Autodesk Inventor part; units mm, degrees
(part 2 of 2)
sketch "Boceto3" plane through (0, 2, 0) normal (0, 1, 0) x (1, 0, 0)
  line L0 (35.7041, 64.3419) -> (35.7041, 63.6919)
  line L1 (35.7042, 59.1622) -> (35.7042, 59.8122)
  line L2 (37.6679, 61.7621) -> (37.6747, 62.4121)
  line L3 (37.6747, 62.4121) -> (38.9746, 62.3985)
  line L4 (37.6679, 61.7621) -> (37.6612, 61.1121)
  line L5 (37.6612, 61.1121) -> (38.961, 61.0986)
  line L6 (41.5539, 61.0919) -> (42.8539, 61.0919) construction
  line L7 (42.8539, 61.0919) -> (42.8539, 58.4716) construction
  spline S0 degree 2 poles (41.5539, 61.0919) (42.8539, 61.0919) (42.8539, 58.4716) knots 1 1 1 2 2 2
  line L8 (41.554, 62.3716) -> (44.1539, 62.3716) construction
  line L9 (44.1539, 62.3716) -> (44.1539, 58.4716) construction
  spline S1 degree 2 poles (41.554, 62.3716) (44.1539, 62.3716) (44.1539, 58.4716) knots 1 1 1 2 2 2
  line L10 (38.954, 61.0919) -> (41.554, 61.0919)
  line L11 (38.9541, 62.3919) -> (41.554, 62.3716)
  line L12 (37.6542, 60.4419) -> (35.7042, 60.4622)
  line L13 (37.6813, 63.0419) -> (35.7041, 63.0419)
  line L14 (37.6813, 63.0419) -> (37.6747, 62.4121)
  line L15 (37.6612, 61.1121) -> (37.6542, 60.4419)
  line L16 (42.8539, 57.8216) -> (44.1539, 57.8216)
  line L17 (44.1539, 57.8216) -> (44.1539, 58.4716)
  line L18 (44.1539, 57.8216) -> (43.8939, 57.8216)
  line L19 (42.8539, 58.4716) -> (42.8539, 57.8216)
  line L20 (58.9613, 57.27) -> (63.5735, 61.1094)
  line L21 (64.2117, 60.8104) -> (64.2117, 53.2631)
  line L22 (58.9754, 56.8292) -> (63.5531, 52.9999)
  arc A0 (63.5531, 52.9999) -> (64.2117, 53.2631) centre (63.7962, 53.3472) ccw
  arc A1 (64.2117, 60.8104) -> (63.5735, 61.1094) centre (63.7975, 60.7568) ccw
  arc A2 (58.9613, 57.27) -> (58.9754, 56.8292) centre (59.2258, 57.0578) ccw
  line L23 (64.4328, 57.3171) -> (69.0449, 61.1564)
  line L24 (69.6831, 60.8575) -> (69.6831, 53.3101)
  line L25 (64.4468, 56.8762) -> (69.0245, 53.0469)
  arc A3 (69.0245, 53.0469) -> (69.6831, 53.3101) centre (69.2676, 53.3943) ccw
  arc A4 (69.6831, 60.8575) -> (69.0449, 61.1564) centre (69.2689, 60.8039) ccw
  arc A5 (64.4328, 57.3171) -> (64.4468, 56.8762) centre (64.6972, 57.1049) ccw
  line L26 (58.9613, 57.27) -> (63.5735, 61.1094)
  line L27 (64.2117, 60.8104) -> (64.2117, 53.2631)
  line L28 (58.9754, 56.8292) -> (63.5531, 52.9999)
  arc A6 (58.9613, 57.27) -> (58.9754, 56.8292) centre (59.2258, 57.0578) ccw
  line L29 (69.6831, 60.8575) -> (69.6831, 53.3101)
  line L30 (64.4328, 57.3171) -> (69.0449, 61.1564)
  line L31 (64.4468, 56.8762) -> (69.0245, 53.0469)
  arc A7 (64.4328, 57.3171) -> (64.4468, 56.8762) centre (64.6972, 57.1049) ccw
  line L32 (128.7561, 56.7254) -> (133.3696, 60.5658)
  line L33 (134.0065, 60.2673) -> (134.0065, 52.7184)
  line L34 (128.7702, 56.2845) -> (133.3479, 52.4552)
  arc A8 (133.3479, 52.4552) -> (134.0065, 52.7184) centre (133.591, 52.8025) ccw
  arc A9 (128.7561, 56.7254) -> (128.7702, 56.2845) centre (129.0205, 56.5132) ccw
  line L35 (139.4779, 60.3128) -> (139.4779, 52.7655)
  arc A10 (138.8193, 52.5023) -> (139.4779, 52.7655) centre (139.0624, 52.8496) ccw
  line L36 (134.2275, 56.7724) -> (138.8397, 60.6118)
  line L37 (134.2416, 56.3316) -> (138.8193, 52.5023)
  arc A11 (134.2275, 56.7724) -> (134.2416, 56.3316) centre (134.4919, 56.5602) ccw
  arc A12 (134.0065, 60.2673) -> (133.3696, 60.5658) centre (133.618, 60.2673) ccw
  arc A13 (139.4779, 60.3128) -> (138.8397, 60.6118) centre (139.0799, 60.294) ccw
  arc A14 (101.959, 62.5573) -> (101.9701, 63.0852) centre (105.955, 62.7371) ccw
  spline S2 degree 3 poles (101.9701, 63.0852) (100.3787, 62.5265) (98.8474, 62.1955) (96.8436, 62.2447) knots 0 0 0 0 1 1 1 1
  circle A15 centre (105.955, 62.7371) radius 1
  arc A16 (108.9509, 62.8921) -> (106.5532, 65.6768) centre (105.955, 62.7371) ccw
  line L38 (109.0736, 62.5385) -> (108.7201, 62.8921)
  line L39 (109.0736, 62.5385) -> (109.4272, 62.8921)
  arc A17 (109.2013, 62.8921) -> (106.5532, 65.9316) centre (105.955, 62.7371) ccw
  line L40 (109.4272, 62.8921) -> (109.2013, 62.8921)
  line L41 (108.9509, 62.8921) -> (108.7201, 62.8921)
  line L42 (102.8865, 63.4069) -> (101.0538, 62.7635) construction
  arc A18 (101.233, 62.841) -> (102.6982, 63.3554) centre (94.7176, 83.7432) ccw construction
  line L43 (96.8436, 62.2447) -> (97.002, 61.7463)
  line L44 (106.5532, 65.9316) -> (106.5532, 65.6768)
  line L45 (35.7041, 64.3419) -> (35.7041, 64.4719)
  line L46 (35.7041, 64.3419) -> (35.7041, 65.6419)
  line L47 (35.7041, 65.6419) -> (33.7541, 65.6419)
  line L48 (33.7541, 65.6419) -> (33.7541, 64.3419)
  line L49 (33.7541, 64.3419) -> (22.7041, 64.3419)
  line L50 (22.7041, 59.1419) -> (22.7041, 64.3419)
  line L51 (33.7541, 59.1419) -> (33.7541, 57.8419)
  line L52 (33.7541, 57.8419) -> (35.704, 57.8419)
  line L53 (35.7042, 57.8419) -> (35.7042, 59.1622)
  line L54 (33.7541, 59.1419) -> (22.7041, 59.1419)
  line L55 (103.5, 23.3722) -> (103.5, 22.8472)
  line L56 (103.5, 19.1886) -> (103.5, 19.7136)
  line L57 (105.0751, 20.2386) -> (103.5, 20.2386)
  line L58 (105.075, 22.3222) -> (103.5, 22.3222)
  line L59 (105.075, 22.3222) -> (105.075, 21.83)
  line L60 (105.0751, 20.78) -> (105.0751, 20.2386)
  line L61 (103.5, 23.3722) -> (103.5, 23.4772)
  line L62 (103.5, 23.3722) -> (103.5, 24.4222)
  line L63 (103.5, 24.4222) -> (101.925, 24.4222)
  line L64 (101.925, 24.4222) -> (101.925, 23.3722)
  line L65 (101.925, 23.3722) -> (93, 23.3722)
  line L66 (93, 19.1722) -> (93, 23.3722)
  line L67 (101.925, 19.1722) -> (101.925, 18.1222)
  line L68 (101.925, 18.1222) -> (103.5, 18.1222)
  line L69 (103.5, 18.1222) -> (103.5, 19.1886)
  line L70 (101.925, 19.1722) -> (93, 19.1722)
  line L71 (103.5, 20.2386) -> (103.5, 19.7136)
  line L72 (103.5, 22.3222) -> (103.5, 22.8472)
  line L73 (35.7042, 60.4622) -> (35.7042, 59.8122)
  line L74 (35.7041, 63.6919) -> (35.7041, 63.0419)
  line L75 (105.075, 21.605) -> (104.7751, 21.605)
  line L76 (104.7751, 21.605) -> (104.7751, 21.005)
  line L77 (104.7751, 21.005) -> (105.0751, 21.005)
  line L78 (105.0751, 21.005) -> (105.0751, 20.78)
  line L79 (105.075, 21.83) -> (105.075, 21.605)
  line L80 (67.3453, 22.5754) -> (66.2953, 22.5754)
  line L81 (66.2953, 22.5754) -> (66.2953, 21.8754)
  line L82 (67.3453, 21.8754) -> (67.3453, 22.5754)
  line L83 (67.3453, 21.8754) -> (67.3453, 21.9454)
  line L84 (67.3453, 21.8754) -> (67.3453, 21.5254)
  line L85 (68.3953, 21.1754) -> (67.3453, 21.1754)
  line L86 (68.3953, 19.7739) -> (67.3453, 19.7754)
  line L87 (67.3453, 19.0754) -> (67.3453, 19.4254)
  line L88 (67.3453, 18.3644) -> (67.3453, 19.0754)
  line L89 (66.2953, 19.074) -> (66.2953, 18.374)
  line L90 (66.2953, 18.374) -> (67.3453, 18.374)
  line L91 (68.3953, 20.1348) -> (68.3953, 19.7739)
  line L92 (67.3453, 19.7754) -> (67.3453, 19.4254)
  line L93 (67.3453, 21.1754) -> (67.3453, 21.5254)
  line L94 (68.3953, 20.2848) -> (68.3953, 20.1348)
  line L95 (68.3953, 21.1754) -> (68.3953, 20.7869)
  line L96 (65.2366, 21.874) -> (65.2366, 19.074)
  line L97 (65.2366, 21.8754) -> (66.2953, 21.8754)
  line L98 (65.2366, 19.074) -> (66.2953, 19.074)
  line L99 (122.2298, 31.1299) -> (122.2298, 16.1299)
  line L100 (122.2298, 16.1299) -> (113.2298, 16.1299)
  line L101 (121.2298, 25.6299) -> (121.2298, 21.6299)
  circle A19 centre (120.4673, 19.4799) radius 0.45
  circle A20 centre (118.8673, 19.4799) radius 0.45
  circle A21 centre (117.2673, 19.4799) radius 0.45
  circle A22 centre (118.8673, 24.2799) radius 0.45
  circle A23 centre (120.4673, 24.2799) radius 0.45
  circle A24 centre (117.2673, 24.2799) radius 0.45
  circle A25 centre (118.8673, 29.0799) radius 0.45
  circle A26 centre (120.4673, 29.0799) radius 0.45
  circle A27 centre (117.2673, 29.0799) radius 0.45
  line L102 (114.9823, 17.6299) -> (117.0198, 17.6299)
  line L103 (117.0198, 17.6299) -> (117.0198, 18.1299)
  line L104 (117.0198, 18.1299) -> (114.9823, 18.1299)
  line L105 (114.9823, 18.1299) -> (114.9823, 17.6299)
  line L106 (114.9823, 22.6299) -> (114.9823, 22.1299)
  line L107 (114.9823, 22.1299) -> (117.0198, 22.1299)
  line L108 (117.0198, 22.6299) -> (114.9823, 22.6299)
  line L109 (117.0198, 22.1299) -> (117.0198, 22.6299)
  line L110 (114.9823, 27.6299) -> (114.9823, 27.1299)
  line L111 (117.0198, 27.6299) -> (114.9823, 27.6299)
  line L112 (117.0198, 27.1299) -> (117.0198, 27.6299)
  line L113 (114.9823, 27.1299) -> (117.0198, 27.1299)
  line L114 (121.2298, 30.6299) -> (121.2298, 26.6299)
  line L115 (93, 23.3722) -> (93, 19.1722)
  line L116 (101.925, 19.1722) -> (93, 19.1722)
  line L117 (101.925, 19.1722) -> (101.925, 18.1222)
  line L118 (101.925, 18.1222) -> (103.5, 18.1222)
  line L119 (103.5, 18.1222) -> (103.5, 20.2386)
  line L120 (103.5, 20.2386) -> (105.0751, 20.2386)
  line L121 (105.0751, 20.2386) -> (105.0751, 21.005)
  line L122 (105.0751, 21.005) -> (104.7751, 21.005)
  line L123 (104.7751, 21.005) -> (104.7751, 21.6108)
  line L124 (104.7751, 21.6108) -> (105.075, 21.6108)
  line L125 (105.075, 21.6108) -> (105.075, 22.3218)
  line L126 (105.075, 22.3218) -> (103.5, 22.3218)
  line L127 (103.5, 22.3218) -> (103.5, 24.4222)
  line L128 (101.925, 24.4222) -> (103.5, 24.4222)
  line L129 (101.925, 24.4222) -> (101.925, 23.3722)
  line L130 (101.925, 23.3722) -> (93, 23.3722)
  line L131 (93, 23.3722) -> (93, 19.1722)
  line L132 (22.7041, 64.3419) -> (22.7041, 59.1419)
  line L133 (22.7041, 59.1419) -> (33.7541, 59.1419)
  line L134 (33.7541, 57.8419) -> (33.7541, 59.1419)
  line L135 (33.7541, 57.8419) -> (35.7042, 57.8419)
  line L136 (35.7042, 57.8419) -> (35.7042, 60.4622)
  line L137 (35.7042, 60.4622) -> (37.6542, 60.4419)
  line L138 (37.6542, 60.4419) -> (37.6612, 61.1121)
  line L139 (37.6612, 61.1121) -> (37.6813, 63.0419)
  line L140 (37.6813, 63.0419) -> (35.7041, 63.0419)
  line L141 (35.7041, 63.0419) -> (35.7041, 65.6419)
  line L142 (35.7041, 65.6419) -> (33.7541, 65.6419)
  line L143 (33.7541, 65.6419) -> (33.7541, 64.3419)
  line L144 (33.7541, 64.3419) -> (22.7041, 64.3419)
  line L145 (22.7041, 64.3419) -> (22.7041, 59.1419)
  line L146 (42.8539, 57.8216) -> (44.1539, 57.8216)
  line L147 (44.1539, 58.4716) -> (44.1539, 57.8216)
  line L148 (42.8539, 58.4716) -> (42.8539, 57.8216)
  line L149 (41.554, 61.0919) -> (42.8539, 61.0919) construction
  line L150 (42.8539, 61.0919) -> (42.8539, 58.4716) construction
  spline S3 degree 2 poles (41.554, 61.0919) (42.8539, 61.0919) (42.8539, 58.4716) knots 1 1 1 2 2 2
  line L151 (41.554, 62.3716) -> (44.1539, 62.3716) construction
  line L152 (44.1539, 62.3716) -> (44.1539, 58.4716) construction
  spline S4 degree 2 poles (41.554, 62.3716) (44.1539, 62.3716) (44.1539, 58.4716) knots 1 1 1 2 2 2
  line L153 (65.2366, 21.8754) -> (65.2366, 19.074)
  line L154 (66.2953, 19.074) -> (65.2366, 19.074)
  line L155 (66.2953, 19.074) -> (66.2953, 18.374)
  line L156 (66.2953, 18.374) -> (67.3453, 18.374)
  line L157 (67.3453, 18.374) -> (67.3453, 19.7754)
  line L158 (67.3453, 19.7754) -> (68.3953, 19.7739)
  line L159 (68.3953, 20.2848) -> (68.3953, 19.7739)
  line L160 (68.3953, 20.7869) -> (68.3953, 21.1754)
  line L161 (68.3953, 21.1754) -> (67.3453, 21.1754)
  line L162 (67.3453, 21.1754) -> (67.3453, 22.5754)
  line L163 (67.3453, 22.5754) -> (66.2953, 22.5754)
  line L164 (66.2953, 22.5754) -> (66.2953, 21.8754)
  line L165 (66.2953, 21.8754) -> (65.2366, 21.8754)
  line L166 (65.2366, 21.8754) -> (65.2366, 19.074)
  spline S5 degree 3 poles (68.3953, 20.7869) (70.7302, 20.7869) (70.1195, 19.8449) (75.3333, 20.4912) knots 0 0 0 0 1 1 1 1
  line L167 (75.3826, 20.0942) -> (75.3333, 20.4912)
  line L168 (37.6612, 61.1121) -> (37.6747, 62.4121)
  line L169 (68.3953, 20.7869) -> (68.3953, 20.3869)
  line L170 (68.3953, 20.3869) -> (68.3953, 19.7739)
  spline S6 degree 5 poles (101.959, 62.5573) (101.0032, 62.2311) (100.0282, 61.9607) (99.0227, 61.7938) (98.0118, 61.7321) (97.002, 61.7463) knots 0 0 0 0 0 0 1 1 1 1 1 1
  spline S7 degree 5 poles (68.3953, 20.3869) (68.7148, 20.3865) (69.0335, 20.3723) (69.3538, 20.3351) (70.0078, 20.1752) (70.6572, 19.9971) (71.008, 19.9385) (72.093, 19.8242) (73.1869, 19.8709) (73.9194, 19.9265) (74.6524, 20.0038) (75.3826, 20.0942) knots 0 0 0 0 0 0 0.226631 0.226631 0.226631 0.477723 0.477723 0.477723 1 1 1 1 1 1
  point P0 (0, 0)
  point P1 (126.2308, 70)
  point P2 (69.853, 20.6217)
  point P3 (70.8385, 20.3864)
  point P4 (117.6798, 19.4799)
  point P5 (117.6798, 24.2799)
  point P6 (117.6798, 29.0799)
  dimension "d288" = 0.4
  dimension "d259" = 1.6
  dimension "d266" = 4.8
  dimension "d276" = 4.5
  dimension "d283" = 5
  constraints: 326 end point, 39 vertical, 36 collinear, 35 point on circle, 28 centre point, 27 perpendicular, 8 horizontal, 6 point on line, 5 coincident, 2 midpoint, 2 parallel, 1 tangent, 64 other
  measures "d259" distance of A19.centre A20.centre
  measures "d266" distance of A21.centre A24.centre
  measures "d276" distance of L102.start L106.end
  measures "d283" distance of L106.start L110.start
extrude "Extrusión15" cut sketch "Boceto3" against normal blind 0.75 contours L0 L74 L13 L14 L2 L4 L15 L12 L73 L1 L53 L52 L51 L54 L50 L49 L48 L47 L46 L45 | L20 A1 L21 A0 L22 A2 | L23 A4 L24 A3 L25 A5 | L32 A12 L33 A8 L34 A9 | L35 A10 L37 A11 L36 A13 | S6 L43 S2 A14 | L55 L72 L58 L59 L79 L124 L123 L76 L77 L78 L60 L57 L71 L56 L69 L68 L67 L70 L66 L65 L64 L63 L62 L61 | L82 L84 L93 L85 L95 L169 L170 L94 L91 L86 L92 L87 L88 L90 L89 L98 L96 L97 L81 L80 | S5 L167 S7 L169
extrude "Extrusión16" cut sketch "Boceto2" against normal blind 4 contours A0 | A1 | L9 L10 L11 L12 L13 | L14 L18 L15 L16 L17 | A2 | A3
extrude "Extrusión17" cut sketch "Boceto8" against normal blind 0.75 contours S28 S29 L13 S37 | L14 L10 S34 S33 S38 S41 S40 S39 S37 | L13 S29 L12 S32 L10 L14 | L10 S35 S36 S34 L14 | S29 S31 S30 S32 L12 | S34 L14 | S40 S41 picked at (114.8488, 38.4188)
extrude "Extrusión18" cut sketch "Boceto6" against normal blind 0.75 contours S0 L3 L4 S10 S9 S5 S8 S6 S7 | S0 S1 S2 L2 | L2 S2 L1 S11 L4 L3 | L4 S3 S4 S10 L3 | S2 S13 S12 S11 L1
